Bottom Connector (Autodesk Fusion 360 archive; units mm, degrees)
design "Hexagon Regular Nut ISO 4032 - M3 Steel 6 Plain"
description: Hexagon Regular Nut ISO 4032 - M3
part number: ISO 4032 - M3 Steel 6 Plain
Autodesk Fusion 360 part; units mm, degrees
sketch "Sketch1" plane through (0, 0, 0) normal (0, 1, 0) x (1, 0, 0)
  line L0 (0, 0) -> (0, -2.4)
  line L1 (-1.5, 0) -> (-2.695, 0)
  line L2 (-2.695, 0) -> (-3.1763, -0.2778)
  line L3 (-3.1763, -0.2778) -> (-3.1763, -2.1222)
  line L4 (-3.1763, -2.1222) -> (-2.695, -2.4)
  line L5 (-2.695, -2.4) -> (-1.5, -2.4)
  line L6 (-1.5, -2.4) -> (-1.5, 0)
  dimension "d121" = 3
  dimension "d122" = 30
  dimension "d123" = 30
  dimension "d128" = 6.3525
  dimension "d172" = 5.39
  dimension "d179" = 2.4
  constraint vertical L0
  constraint coincident L0 L0.end
  constraint coincident origin L0
  constraint horizontal L1
  constraint coincident L0.start L1
  constraint coincident L0.start origin
  constraint coincident L0.end L5
  constraint vertical L1.end L4.end
  measures "d122" angle of L1 L2
  measures "d123" angle of L4 L5
  measures "d179" distance of L1 L5
revolve "Revolve1" add sketch "Sketch1" angle 360 about axis through (0, 0, 0) along (0, 0, 1)
sketch "Sketch8" plane through (0, 0, 2.4) normal (0, 0, 1) x (1, 0, 0)
  line L0 (-2.75, -1.5894) -> (-2.75, 1.5894)
  circle A0 centre (0, 0) radius 1.5
  circle A1 centre (0, 0) radius 3.1763
  dimension "d114" = 2.75
  constraint coincident L0.end A1
  constraint coincident L0.start A1
  constraint vertical L0
  measures "d114" distance of A0.centre L0
extrude "Extrude5" cut sketch "Sketch8" against normal blind 2.4 contours L0 A1 picked at (-2.8188, -0.3871)
pattern_circular "C-Pattern2" count 6 over 360 about axis through (0, 0, 1.75) along (0, 0, 1) of "Extrude5"
thread "Thread3" "ISO Metric profile 3.0 M3x0.5 M3x0.5 6H" major diameter 3.086 minor diameter 2.529 pitch 0.5 angle 60 resizes the face on face at (-1.4925, 0.1494, 1.6)
sketch "Sketch12" plane through (0, 0, 0) normal (0, 1, 0) x (1, 0, 0)
  line L0 (-1.5, 0) -> (0, 0)
  line L1 (-0.8072, -1.2) -> (-1.5, 0)
  line L2 (-1.5, -2.4) -> (0, -2.4)
  line L3 (-0.8072, -1.2) -> (-1.5, -2.4)
  line L4 (0, 0) -> (0, -2.4)
  dimension "d169" = 60
  dimension "d177" = 1.5
  dimension "d178" = 60
  constraint horizontal L0
  constraint coincident L1.start L3.start
  constraint vertical L0.start L2.start
  constraint coincident L2.end L4.end
  constraint coincident L0.end L4.start
  constraint perpendicular L2 L4
  measures "d169" angle of L2 L3
  measures "d177" distance of L0.start L4
  measures "d178" angle of L0 L1
revolve "Revolve3" cut sketch "Sketch12" angle 360 about axis through (0, 0, 1.75) along (0, 0, 1)
equation "adsk_nheig = 2.40 mm"
equation "adsk_maxdia = 6.3525 mm"
equation "adsk_nomdia = 3.00 mm"
equation "d89 = -adsk_nheig"
equation "adsk_waflat = 5.50 mm"
equation "d114 = adsk_waflat / 2"
equation "adsk_chamang1 = 30.00 deg"
equation "adsk_chamang2 = 30.00 deg"
equation "d121 = adsk_nomdia"
equation "d122 = adsk_chamang1"
equation "d123 = adsk_chamang2"
equation "d128 = adsk_maxdia"
equation "d163 = adsk_nheig"
equation "adsk_beardia = 5.39 mm"
equation "d172 = adsk_beardia"
equation "d177 = adsk_nomdia * 0.5"
equation "d179 = adsk_nheig"

design "Bottom Connector" references "Bottom Connector", "M3 Nut"
part number: 2026-01-14-14-46-55-393
Autodesk Fusion 360 part; units mm, degrees
sketch "Base" plane through (0, 0, 0) normal (0, 0, 1) x (1, 0, 0)
  line L0 (12, 5) -> (-12, 5)
  line L1 (-12, 5) -> (-12, -5)
  line L2 (-12, -5) -> (12, -5)
  line L3 (12, -5) -> (12, 5)
  line L4 (12, 5) -> (-12, -5) construction
  line L5 (-12, 5) -> (12, -5) construction
  circle A0 centre (6, 0) radius 1.65
  circle A1 centre (-6, 0) radius 1.65
  dimension "d110" = 24
  dimension "d111" = 10
  dimension "d112" = 3.3
  dimension "d113" = 3.3
  constraint horizontal L0
  constraint perpendicular L0 L1
  constraint parallel L0 L2
  constraint parallel L1 L3
  constraint coincident L4 origin
  constraint coincident L5 origin
  measures "d110" distance of L1.end L2.end
  measures "d111" distance of L0.end L1.end
  measures "d112" diameter of A0
  measures "d113" diameter of A1
extrude "Extrude27" add sketch "Base" along normal blind 0.5
sketch "Nut Holders" plane through (0, 0, 0) normal (0, 0, 1) x (1, 0, 0)
  line L0 (-12, 5, 0.5) -> (12, 5, 0.5)
  line L1 (12, 5, 0.5) -> (12, -5, 0.5)
  line L2 (12, -5, 0.5) -> (-12, -5, 0.5)
  line L3 (-12, -5, 0.5) -> (-12, 5, 0.5)
  line L4 (-3.25, 1.6166, 0.5) -> (-6.05, 3.2332, 0.5)
  line L5 (-6.05, 3.2332, 0.5) -> (-8.85, 1.6166, 0.5)
  line L6 (-8.85, 1.6166, 0.5) -> (-8.85, -1.6166, 0.5)
  line L7 (-8.85, -1.6166, 0.5) -> (-6.05, -3.2332, 0.5)
  line L8 (-6.05, -3.2332, 0.5) -> (-3.25, -1.6166, 0.5)
  line L9 (-3.25, -1.6166, 0.5) -> (-3.25, 1.6166, 0.5)
  line L10 (8.75, 1.6166, 0.5) -> (5.95, 3.2332, 0.5)
  line L11 (5.95, 3.2332, 0.5) -> (3.15, 1.6166, 0.5)
  line L12 (3.15, 1.6166, 0.5) -> (3.15, -1.6166, 0.5)
  line L13 (3.15, -1.6166, 0.5) -> (5.95, -3.2332, 0.5)
  line L14 (5.95, -3.2332, 0.5) -> (8.75, -1.6166, 0.5)
  line L15 (8.75, -1.6166, 0.5) -> (8.75, 1.6166, 0.5)
  point P0 (-6.05, 0)
  point P1 (5.95, 0)
  dimension "d116" = 2.8
  dimension "d117" = 2.8
extrude "Extrude28" add sketch "Nut Holders" along normal blind 2.5 contours L0 L1 L2 L3 in plane through (0, 0, 0.5) normal (0, 0, 1)
extrude "Extrude29" cut 1 faces at (-8.45, 0, 0.5) along direction (0, 0, -1) blind 0.1
extrude "Extrude30" cut 1 faces at (3.55, 0, 0.5) along direction (0, 0, -1) blind 0.1
extrude "Extrude31" cut 1 faces at (-10.55, 0, 0) along direction (0, 0, 1) blind 0.2
move_body "Move12" bodies 1 to x (1, 0, 0) y (0, 1, 0) z (0, 0, 1) at (0, 0, -0.2)
